Autodesk Fusion 360 part; units mm, degrees
(part 2 of 7)
sketch "Sketch40" plane through (0, 116.2145, -31.1396) normal (0, 0.965926, -0.258819) x (-1, 0, 0)
  line L0 (-109.8689, 117.075) -> (-111.5449, 117.075)
  arc A0 (-116.5449, 122.075) -> (-111.5449, 117.075) centre (-111.5449, 122.075) ccw
  line L1 (-116.5449, 122.075) -> (-116.5449, 197.0502)
  arc A1 (-111.5449, 202.0502) -> (-116.5449, 197.0502) centre (-111.5449, 197.0502) ccw
  line L2 (-111.5449, 202.0502) -> (-109.8689, 202.0502)
  arc A2 (-104.8689, 197.0502) -> (-109.8689, 202.0502) centre (-109.8689, 197.0502) ccw
  line L3 (-104.8689, 197.0502) -> (-104.8689, 122.075)
  arc A3 (-109.8689, 117.075) -> (-104.8689, 122.075) centre (-109.8689, 122.075) ccw
  line L4 (-35, 125) -> (-35, 117.5)
  arc A4 (-37.5, 115) -> (-35, 117.5) centre (-37.5, 117.5) ccw
  line L5 (-37.5, 115) -> (-65, 115)
  arc A5 (-70, 120) -> (-65, 115) centre (-65, 120) ccw
  line L6 (-70, 120) -> (-70, 125)
  arc A6 (-65, 130) -> (-70, 125) centre (-65, 125) ccw
  line L7 (-65, 130) -> (-40, 130)
  arc A7 (-35, 125) -> (-40, 130) centre (-40, 125) ccw
  line L8 (-95.5983, 117.0948) -> (-95.6526, 117.0948)
  arc A8 (-100.6526, 122.0948) -> (-95.6526, 117.0948) centre (-95.6526, 122.0948) ccw
  line L9 (-100.6526, 122.0948) -> (-100.6526, 154.3733)
  line L10 (-100.6526, 154.3733) -> (-90.5983, 154.3733)
  line L11 (-90.5983, 154.3733) -> (-90.5983, 122.0948)
  arc A9 (-95.5983, 117.0948) -> (-90.5983, 122.0948) centre (-95.5983, 122.0948) ccw
  arc A10 (-90.5983, 197.0502) -> (-95.5983, 202.0502) centre (-95.5983, 197.0502) ccw
  line L12 (-90.5983, 197.0502) -> (-90.5983, 159.5626)
  line L13 (-90.5983, 159.5626) -> (-100.6526, 159.5626)
  line L14 (-100.6526, 159.5626) -> (-100.6526, 197.0502)
  arc A11 (-95.6526, 202.0502) -> (-100.6526, 197.0502) centre (-95.6526, 197.0502) ccw
  line L15 (-95.6526, 202.0502) -> (-95.5983, 202.0502)
  line L16 (-37.5, 135) -> (-67.5, 135)
  arc A12 (-70, 137.5) -> (-67.5, 135) centre (-67.5, 137.5) ccw
  line L17 (-70, 137.5) -> (-70, 142.5)
  arc A13 (-67.5, 145) -> (-70, 142.5) centre (-67.5, 142.5) ccw
  line L18 (-67.5, 145) -> (-37.5, 145)
  arc A14 (-35, 142.5) -> (-37.5, 145) centre (-37.5, 142.5) ccw
  line L19 (-35, 142.5) -> (-35, 137.5)
  arc A15 (-37.5, 135) -> (-35, 137.5) centre (-37.5, 137.5) ccw
  arc A16 (-84.2974, 121.8844) -> (-80.3534, 116.9972) centre (-79.2974, 121.8844) ccw
  line L20 (-84.2974, 121.8844) -> (-84.2974, 171.0352)
  line L21 (-84.2974, 171.0352) -> (-76.4093, 171.0352)
  line L22 (-76.4093, 171.0352) -> (-76.4093, 121.8844)
  arc A17 (-80.3534, 116.9972) -> (-76.4093, 121.8844) centre (-81.4093, 121.8844) ccw
  arc A18 (-76.4093, 196.948) -> (-80.3534, 201.8353) centre (-81.4093, 196.948) ccw
  line L23 (-76.4093, 196.948) -> (-76.4093, 176.5782)
  line L24 (-76.4093, 176.5782) -> (-84.2974, 176.5782)
  line L25 (-84.2974, 176.5782) -> (-84.2974, 196.948)
  arc A19 (-80.3534, 201.8353) -> (-84.2974, 196.948) centre (-79.2974, 196.948) ccw
  line L26 (-120, 85) -> (-120, 100)
  arc A20 (-110, 110) -> (-120, 100) centre (-110, 100) ccw
  line L27 (-110, 110) -> (-61.6636, 110)
  arc A21 (-51.6636, 100) -> (-61.6636, 110) centre (-61.6636, 100) ccw
  line L28 (-51.6636, 100) -> (-51.6636, 85)
  arc A22 (-61.6636, 75) -> (-51.6636, 85) centre (-61.6636, 85) ccw
  line L29 (-61.6636, 75) -> (-110, 75)
  arc A23 (-120, 85) -> (-110, 75) centre (-110, 85) ccw
  line L30 (-45.44, 85) -> (-45.44, 100)
  arc A24 (-35.44, 110) -> (-45.44, 100) centre (-35.44, 100) ccw
  line L31 (-35.44, 110) -> (-20, 110)
  arc A25 (-10, 100) -> (-20, 110) centre (-20, 100) ccw
  line L32 (-10, 100) -> (-10, 85)
  arc A26 (-20, 75) -> (-10, 85) centre (-20, 85) ccw
  line L33 (-20, 75) -> (-35.44, 75)
  arc A27 (-45.44, 85) -> (-35.44, 75) centre (-35.44, 85) ccw
  line L34 (22.9316, 100) -> (22.9316, 85)
  arc A28 (12.9316, 75) -> (22.9316, 85) centre (12.9316, 85) ccw
  line L35 (12.9316, 75) -> (7.9281, 75)
  arc A29 (-2.0719, 85) -> (7.9281, 75) centre (7.9281, 85) ccw
  line L36 (-2.0719, 85) -> (-2.0719, 100)
  arc A30 (7.9281, 110) -> (-2.0719, 100) centre (7.9281, 100) ccw
  line L37 (7.9281, 110) -> (12.9316, 110)
  arc A31 (22.9316, 100) -> (12.9316, 110) centre (12.9316, 100) ccw
  line L38 (-40, 30) -> (-110, 30)
  arc A32 (-120, 40) -> (-110, 30) centre (-110, 40) ccw
  line L39 (-120, 40) -> (-120, 60)
  arc A33 (-110, 70) -> (-120, 60) centre (-110, 60) ccw
  line L40 (-110, 70) -> (-40, 70)
  arc A34 (-30, 60) -> (-40, 70) centre (-40, 60) ccw
  line L41 (-30, 60) -> (-30, 40)
  arc A35 (-40, 30) -> (-30, 40) centre (-40, 40) ccw
  line L42 (-10, 70) -> (10, 70)
  arc A36 (20, 60) -> (10, 70) centre (10, 60) ccw
  line L43 (20, 60) -> (20, 40)
  arc A37 (10, 30) -> (20, 40) centre (10, 40) ccw
  line L44 (10, 30) -> (-10, 30)
  arc A38 (-20, 40) -> (-10, 30) centre (-10, 40) ccw
  line L45 (-20, 40) -> (-20, 60)
  arc A39 (-10, 70) -> (-20, 60) centre (-10, 60) ccw
  ellipse E0 centre (22.741, -39.3535) end of major axis (22.741, -46.5838) minor radius 7 (22.741, -46.5838) -> (29.741, -39.3535) ccw
  line L46 (29.741, -39.3535) -> (29.741, 209.5755)
  ellipse E1 centre (22.741, 209.5755) end of major axis (22.741, 216.8058) minor radius 7 (29.741, 209.5755) -> (22.741, 216.8058) ccw
  line L47 (22.741, 216.8058) -> (-123.259, 216.8058)
  ellipse E2 centre (-123.259, 209.5755) end of major axis (-123.259, 216.8058) minor radius 7 (-123.259, 216.8058) -> (-130.259, 209.5755) ccw
  line L48 (-130.259, 209.5755) -> (-130.259, -39.3535)
  ellipse E3 centre (-123.259, -39.3535) end of major axis (-123.259, -46.5838) minor radius 7 (-130.259, -39.3535) -> (-123.259, -46.5838) ccw
  line L49 (-123.259, -46.5838) -> (22.741, -46.5838)
  line L50 (-35.9419, 179.9959) -> (-35.9419, 150.9959)
  line L51 (-35.9419, 150.9959) -> (-72.9419, 150.9959)
  line L52 (-72.9419, 150.9959) -> (-72.9419, 179.9959)
  line L53 (-72.9419, 179.9959) -> (-35.9419, 179.9959)
  line L54 (0, 145) -> (25, 155)
  line L55 (25, 155) -> (25, 160)
  line L56 (25, 160) -> (0, 150)
  line L57 (0, 150) -> (0, 145)
  line L58 (0, 155) -> (25, 165)
  line L59 (25, 165) -> (25, 170)
  line L60 (25, 170) -> (0, 160)
  line L61 (0, 160) -> (0, 155)
  line L62 (0, 165) -> (25, 175)
  line L63 (25, 175) -> (25, 180.1705)
  line L64 (0, 165) -> (0, 170)
  line L65 (0, 170) -> (25, 180.1705)
  line L66 (0, 175) -> (25, 185)
  line L67 (25, 185) -> (25, 190.1897)
  line L68 (25, 190.1897) -> (0, 180.1897)
  line L69 (0, 180.1897) -> (0, 175)
  line L70 (0, 185) -> (25, 195)
  line L71 (25, 195) -> (25, 200)
  line L72 (25, 200) -> (0, 190)
  line L73 (0, 190) -> (0, 185)
  line L74 (0, 195) -> (25, 205)
  line L75 (25, 205) -> (25, 210)
  line L76 (25, 210) -> (0, 200)
  line L77 (0, 200) -> (0, 195)
  line L78 (-5, 145) -> (-30, 150)
  line L79 (-30, 150) -> (-30, 155)
  line L80 (-30, 155) -> (-5, 150)
  line L81 (-5, 150) -> (-5, 145)
  line L82 (-5, 155) -> (-30, 160)
  line L83 (-30, 160) -> (-30, 165.149)
  line L84 (-30, 165.149) -> (-5, 160.149)
  line L85 (-5, 160.149) -> (-5, 155)
  line L86 (-5, 165) -> (-30, 170)
  line L87 (-30, 170) -> (-30, 175)
  line L88 (-30, 175) -> (-5, 170)
  line L89 (-5, 170) -> (-5, 165)
  line L90 (-5, 175) -> (-30, 180)
  line L91 (-30, 180) -> (-30, 184.9041)
  line L92 (-30, 184.9041) -> (-5, 180)
  line L93 (-5, 180) -> (-5, 175)
  line L94 (-5, 184.9041) -> (-30, 189.9041)
  line L95 (-30, 189.9041) -> (-30, 195)
  line L96 (-30, 195) -> (-5, 190)
  line L97 (-5, 184.9041) -> (-5, 190)
  line L98 (-5, 195) -> (-30, 200)
  line L99 (-30, 200) -> (-30, 205)
  line L100 (-30, 205) -> (-5, 200)
  line L101 (-5, 200) -> (-5, 195)
  constraint parallel L54 L56
  constraint parallel L56 L58
  constraint parallel L57 L59
  constraint parallel L56 L60
  constraint parallel L57 L61
  constraint parallel L60 L62
  constraint parallel L61 L63
  constraint vertical L64
  constraint parallel L62 L66
  constraint parallel L63 L67
  constraint parallel L62 L68
  constraint vertical L69
  constraint parallel L66 L70
  constraint parallel L69 L71
  constraint parallel L70 L72
  constraint parallel L71 L73
  constraint parallel L72 L74
  constraint parallel L73 L75
  constraint parallel L74 L76
  constraint parallel L75 L77
  constraint parallel L78 L82
  constraint parallel L81 L83
  constraint parallel L78 L84
  constraint parallel L82 L86
  constraint parallel L85 L87
  constraint parallel L82 L88
  constraint parallel L86 L90
  constraint parallel L89 L91
  constraint parallel L90 L94
  constraint parallel L93 L95
  constraint parallel L90 L96
  constraint parallel L96 L98
  constraint parallel L97 L99
  constraint parallel L96 L100
  constraint vertical L101
sketch "Sketch41" plane through (0, 116.2145, -31.1396) normal (0, 0.965926, -0.258819) x (-1, 0, 0)
  line L0 (25, 185) -> (0, 175)
  line L1 (0, 175) -> (0, 180.1897)
  line L2 (0, 180.1897) -> (25, 190.1897)
  line L3 (25, 190.1897) -> (25, 185)
  line L4 (-5, 190) -> (-5, 184.9041)
  line L5 (-5, 184.9041) -> (-30, 189.9041)
  line L6 (-30, 189.9041) -> (-30, 195)
  line L7 (-30, 195) -> (-5, 190)
  line L8 (-30, 150) -> (-30, 155)
  line L9 (-30, 155) -> (-5, 150)
  line L10 (-5, 150) -> (-5, 145)
  line L11 (-5, 145) -> (-30, 150)
  line L12 (-30, 160) -> (-30, 165.149)
  line L13 (-30, 165.149) -> (-5, 160.149)
  line L14 (-5, 160.149) -> (-5, 155)
  line L15 (-5, 155) -> (-30, 160)
  line L16 (-30, 200) -> (-30, 205)
  line L17 (-30, 205) -> (-5, 200)
  line L18 (-5, 200) -> (-5, 195)
  line L19 (-5, 195) -> (-30, 200)
  line L20 (25, 180.1705) -> (25, 175)
  line L21 (25, 175) -> (0, 165)
  line L22 (0, 165) -> (0, 170)
  line L23 (0, 170) -> (25, 180.1705)
  line L24 (25, 155) -> (0, 145)
  line L25 (0, 145) -> (0, 150)
  line L26 (0, 150) -> (25, 160)
  line L27 (25, 160) -> (25, 155)
  line L28 (25, 195) -> (0, 185)
  line L29 (0, 185) -> (0, 190)
  line L30 (0, 190) -> (25, 200)
  line L31 (25, 200) -> (25, 195)
  line L32 (-30, 180) -> (-30, 184.9041)
  line L33 (-30, 184.9041) -> (-5, 180)
  line L34 (-5, 180) -> (-5, 175)
  line L35 (-5, 175) -> (-30, 180)
  line L36 (-30, 170) -> (-30, 175)
  line L37 (-30, 175) -> (-5, 170)
  line L38 (-5, 170) -> (-5, 165)
  line L39 (-5, 165) -> (-30, 170)
  line L40 (25, 205) -> (0, 195)
  line L41 (0, 195) -> (0, 200)
  line L42 (0, 200) -> (25, 210)
  line L43 (25, 210) -> (25, 205)
  line L44 (25, 165) -> (0, 155)
  line L45 (0, 155) -> (0, 160)
  line L46 (0, 160) -> (25, 170)
  line L47 (25, 170) -> (25, 165)
  line L48 (-109.8689, 117.075) -> (-111.5449, 117.075)
  arc A0 (-116.5449, 122.075) -> (-111.5449, 117.075) centre (-111.5449, 122.075) ccw
  line L49 (-116.5449, 122.075) -> (-116.5449, 197.0502)
  arc A1 (-111.5449, 202.0502) -> (-116.5449, 197.0502) centre (-111.5449, 197.0502) ccw
  line L50 (-111.5449, 202.0502) -> (-109.8689, 202.0502)
  arc A2 (-104.8689, 197.0502) -> (-109.8689, 202.0502) centre (-109.8689, 197.0502) ccw
  line L51 (-104.8689, 197.0502) -> (-104.8689, 122.075)
  arc A3 (-109.8689, 117.075) -> (-104.8689, 122.075) centre (-109.8689, 122.075) ccw
  line L52 (-35, 125) -> (-35, 117.5)
  arc A4 (-37.5, 115) -> (-35, 117.5) centre (-37.5, 117.5) ccw
  line L53 (-37.5, 115) -> (-65, 115)
  arc A5 (-70, 120) -> (-65, 115) centre (-65, 120) ccw
  line L54 (-70, 120) -> (-70, 125)
  arc A6 (-65, 130) -> (-70, 125) centre (-65, 125) ccw
  line L55 (-65, 130) -> (-40, 130)
  arc A7 (-35, 125) -> (-40, 130) centre (-40, 125) ccw
  line L56 (-95.5983, 117.0948) -> (-95.6526, 117.0948)
  arc A8 (-100.6526, 122.0948) -> (-95.6526, 117.0948) centre (-95.6526, 122.0948) ccw
  line L57 (-100.6526, 122.0948) -> (-100.6526, 154.3733)
  line L58 (-100.6526, 154.3733) -> (-90.5983, 154.3733)
  line L59 (-90.5983, 154.3733) -> (-90.5983, 122.0948)
  arc A9 (-95.5983, 117.0948) -> (-90.5983, 122.0948) centre (-95.5983, 122.0948) ccw
  arc A10 (-90.5983, 197.0502) -> (-95.5983, 202.0502) centre (-95.5983, 197.0502) ccw
  line L60 (-90.5983, 197.0502) -> (-90.5983, 159.5626)
  line L61 (-90.5983, 159.5626) -> (-100.6526, 159.5626)
  line L62 (-100.6526, 159.5626) -> (-100.6526, 197.0502)
  arc A11 (-95.6526, 202.0502) -> (-100.6526, 197.0502) centre (-95.6526, 197.0502) ccw
  line L63 (-95.6526, 202.0502) -> (-95.5983, 202.0502)
  line L64 (-37.5, 135) -> (-67.5, 135)
  arc A12 (-70, 137.5) -> (-67.5, 135) centre (-67.5, 137.5) ccw
  line L65 (-70, 137.5) -> (-70, 142.5)
  arc A13 (-67.5, 145) -> (-70, 142.5) centre (-67.5, 142.5) ccw
  line L66 (-67.5, 145) -> (-37.5, 145)
  arc A14 (-35, 142.5) -> (-37.5, 145) centre (-37.5, 142.5) ccw
  line L67 (-35, 142.5) -> (-35, 137.5)
  arc A15 (-37.5, 135) -> (-35, 137.5) centre (-37.5, 137.5) ccw
  arc A16 (-84.2974, 121.8844) -> (-80.3534, 116.9972) centre (-79.2974, 121.8844) ccw
  line L68 (-84.2974, 121.8844) -> (-84.2974, 171.0352)
  line L69 (-84.2974, 171.0352) -> (-76.4093, 171.0352)
  line L70 (-76.4093, 171.0352) -> (-76.4093, 121.8844)
  arc A17 (-80.3534, 116.9972) -> (-76.4093, 121.8844) centre (-81.4093, 121.8844) ccw
  arc A18 (-76.4093, 196.948) -> (-80.3534, 201.8353) centre (-81.4093, 196.948) ccw
  line L71 (-76.4093, 196.948) -> (-76.4093, 176.5782)
  line L72 (-76.4093, 176.5782) -> (-84.2974, 176.5782)
  line L73 (-84.2974, 176.5782) -> (-84.2974, 196.948)
  arc A19 (-80.3534, 201.8353) -> (-84.2974, 196.948) centre (-79.2974, 196.948) ccw
  line L74 (-120, 85) -> (-120, 100)
  arc A20 (-110, 110) -> (-120, 100) centre (-110, 100) ccw
  line L75 (-110, 110) -> (-61.6636, 110)
  arc A21 (-51.6636, 100) -> (-61.6636, 110) centre (-61.6636, 100) ccw
  line L76 (-51.6636, 100) -> (-51.6636, 85)
  arc A22 (-61.6636, 75) -> (-51.6636, 85) centre (-61.6636, 85) ccw
  line L77 (-61.6636, 75) -> (-110, 75)
  arc A23 (-120, 85) -> (-110, 75) centre (-110, 85) ccw
  line L78 (-45.44, 85) -> (-45.44, 100)
  arc A24 (-35.44, 110) -> (-45.44, 100) centre (-35.44, 100) ccw
  line L79 (-35.44, 110) -> (-20, 110)
  arc A25 (-10, 100) -> (-20, 110) centre (-20, 100) ccw
  line L80 (-10, 100) -> (-10, 85)
  arc A26 (-20, 75) -> (-10, 85) centre (-20, 85) ccw
  line L81 (-20, 75) -> (-35.44, 75)
  arc A27 (-45.44, 85) -> (-35.44, 75) centre (-35.44, 85) ccw
  line L82 (22.9316, 100) -> (22.9316, 85)
  arc A28 (12.9316, 75) -> (22.9316, 85) centre (12.9316, 85) ccw
  line L83 (12.9316, 75) -> (7.9281, 75)
  arc A29 (-2.0719, 85) -> (7.9281, 75) centre (7.9281, 85) ccw
  line L84 (-2.0719, 85) -> (-2.0719, 100)
  arc A30 (7.9281, 110) -> (-2.0719, 100) centre (7.9281, 100) ccw
  line L85 (7.9281, 110) -> (12.9316, 110)
  arc A31 (22.9316, 100) -> (12.9316, 110) centre (12.9316, 100) ccw
  line L86 (-40, 30) -> (-110, 30)
  arc A32 (-120, 40) -> (-110, 30) centre (-110, 40) ccw
  line L87 (-120, 40) -> (-120, 60)
  arc A33 (-110, 70) -> (-120, 60) centre (-110, 60) ccw
  line L88 (-110, 70) -> (-40, 70)
  arc A34 (-30, 60) -> (-40, 70) centre (-40, 60) ccw
  line L89 (-30, 60) -> (-30, 40)
  arc A35 (-40, 30) -> (-30, 40) centre (-40, 40) ccw
  line L90 (-10, 70) -> (10, 70)
  arc A36 (20, 60) -> (10, 70) centre (10, 60) ccw
  line L91 (20, 60) -> (20, 40)
  arc A37 (10, 30) -> (20, 40) centre (10, 40) ccw
  line L92 (10, 30) -> (-10, 30)
  arc A38 (-20, 40) -> (-10, 30) centre (-10, 40) ccw
  line L93 (-20, 40) -> (-20, 60)
  arc A39 (-10, 70) -> (-20, 60) centre (-10, 60) ccw
  ellipse E0 centre (22.741, -39.3535) end of major axis (22.741, -46.5838) minor radius 7 (22.741, -46.5838) -> (29.741, -39.3535) ccw
  line L94 (29.741, -39.3535) -> (29.741, 209.5755)
  ellipse E1 centre (22.741, 209.5755) end of major axis (22.741, 216.8058) minor radius 7 (29.741, 209.5755) -> (22.741, 216.8058) ccw
  line L95 (22.741, 216.8058) -> (-123.259, 216.8058)
  ellipse E2 centre (-123.259, 209.5755) end of major axis (-123.259, 216.8058) minor radius 7 (-123.259, 216.8058) -> (-130.259, 209.5755) ccw
  line L96 (-130.259, 209.5755) -> (-130.259, -39.3535)
  ellipse E3 centre (-123.259, -39.3535) end of major axis (-123.259, -46.5838) minor radius 7 (-130.259, -39.3535) -> (-123.259, -46.5838) ccw
  line L97 (-123.259, -46.5838) -> (22.741, -46.5838)
  line L98 (-35.9419, 179.9959) -> (-35.9419, 150.9959)
  line L99 (-35.9419, 150.9959) -> (-72.9419, 150.9959)
  line L100 (-72.9419, 150.9959) -> (-72.9419, 179.9959)
  line L101 (-72.9419, 179.9959) -> (-35.9419, 179.9959)
  line L102 (-68.3957, 196.948) -> (-56.6, 196.948)
  line L103 (-55, 195.348) -> (-55, 186.6)
  line L104 (-56.6, 185) -> (-68.3957, 185)
  line L105 (-69.9957, 186.6) -> (-69.9957, 195.348)
  line L106 (-48.311, 196.948) -> (-36.6, 196.948)
  line L107 (-35, 195.348) -> (-35, 186.6)
  line L108 (-36.6, 185) -> (-48.311, 185)
  line L109 (-49.911, 186.6) -> (-49.911, 195.348)
  line L110 (-68.7895, 206.1671) -> (-56.6, 206.1671)
  line L111 (-55, 204.5671) -> (-55, 201.6)
  line L112 (-56.6, 200) -> (-68.7895, 200)
  line L113 (-70.3895, 201.6) -> (-70.3895, 204.5671)
  line L114 (-48.311, 206.2984) -> (-36.6, 206.2984)
  line L115 (-35, 204.6984) -> (-35, 201.6)
  line L116 (-36.6, 200) -> (-48.311, 200)
  line L117 (-49.911, 201.6) -> (-49.911, 204.6984)
  arc A40 (-68.7895, 206.1671) -> (-70.3895, 204.5671) centre (-68.7895, 204.5671) ccw
  arc A41 (-70.3895, 201.6) -> (-68.7895, 200) centre (-68.7895, 201.6) ccw
  arc A42 (-56.6, 200) -> (-55, 201.6) centre (-56.6, 201.6) ccw
  arc A43 (-55, 204.5671) -> (-56.6, 206.1671) centre (-56.6, 204.5671) ccw
  arc A44 (-48.311, 206.2984) -> (-49.911, 204.6984) centre (-48.311, 204.6984) ccw
  arc A45 (-49.911, 201.6) -> (-48.311, 200) centre (-48.311, 201.6) ccw
  arc A46 (-36.6, 200) -> (-35, 201.6) centre (-36.6, 201.6) ccw
  arc A47 (-35, 204.6984) -> (-36.6, 206.2984) centre (-36.6, 204.6984) ccw
  arc A48 (-35, 195.348) -> (-36.6, 196.948) centre (-36.6, 195.348) ccw
  arc A49 (-48.311, 196.948) -> (-49.911, 195.348) centre (-48.311, 195.348) ccw
  arc A50 (-49.911, 186.6) -> (-48.311, 185) centre (-48.311, 186.6) ccw
  arc A51 (-36.6, 185) -> (-35, 186.6) centre (-36.6, 186.6) ccw
  arc A52 (-56.6, 185) -> (-55, 186.6) centre (-56.6, 186.6) ccw
  arc A53 (-69.9957, 186.6) -> (-68.3957, 185) centre (-68.3957, 186.6) ccw
  arc A54 (-68.3957, 196.948) -> (-69.9957, 195.348) centre (-68.3957, 195.348) ccw
  arc A55 (-55, 195.348) -> (-56.6, 196.948) centre (-56.6, 195.348) ccw
  dimension "d130" = 1.6
  constraint horizontal L102
  constraint vertical L103
  constraint horizontal L104
  constraint vertical L105
  constraint horizontal L106
  constraint vertical L107
  constraint horizontal L108
  constraint vertical L109
  constraint horizontal L110
  constraint vertical L111
  constraint horizontal L112
  constraint vertical L113
  constraint horizontal L114
  constraint vertical L115
  constraint horizontal L116
  constraint vertical L117
  constraint tangent L110 A40
  constraint tangent L113 A40
  constraint tangent L112 A41
  constraint tangent L113 A41
  constraint equal A40 A41
  constraint tangent L111 A42
  constraint tangent L112 A42
  constraint equal A40 A42
  constraint tangent L110 A43
  constraint tangent L111 A43
  constraint equal A40 A43
  constraint tangent L114 A44
  constraint tangent L117 A44
  constraint equal A40 A44
  constraint tangent L116 A45
  constraint tangent L117 A45
  constraint equal A40 A45
  constraint tangent L115 A46
  constraint tangent L116 A46
  constraint equal A40 A46
  constraint tangent L114 A47
  constraint tangent L115 A47
  constraint equal A40 A47
  constraint tangent L106 A48
  constraint tangent L107 A48
  constraint equal A40 A48
  constraint tangent L106 A49
  constraint tangent L109 A49
  constraint equal A40 A49
  constraint tangent L108 A50
  constraint tangent L109 A50
  constraint equal A40 A50
  constraint tangent L107 A51
  constraint tangent L108 A51
  constraint equal A40 A51
  constraint tangent L103 A52
  constraint tangent L104 A52
  constraint equal A40 A52
  constraint tangent L104 A53
  constraint tangent L105 A53
  constraint equal A40 A53
  constraint tangent L102 A54
  constraint tangent L105 A54
  constraint equal A40 A54
  constraint tangent L102 A55
  constraint tangent L103 A55
  constraint equal A40 A55
  measures "d130" radius of A40
sketch "Sketch42" plane through (130.259, 0, 0) normal (1, 0, 0) x (0, 0, -1)
  line L0 (-45, 101.218) -> (-45, 110)
  line L1 (-45, 110) -> (-6.7003, 110)
  line L2 (-6.7003, 110) -> (-6.7003, 101.218)
  line L3 (-6.7003, 101.218) -> (-45, 101.218)
  line L4 (69.1009, 100.1665) -> (69.1521, 106.0291)
  line L5 (69.1521, 106.0291) -> (-171.2948, 170.4566)
  line L6 (-171.2948, 170.4566) -> (-171.8899, 102.2696)
  line L7 (-171.8899, 102.2696) -> (69.1009, 100.1665)
  line L8 (-161.2986, 157.4875) -> (-51.9598, 127.9462)
  line L9 (-50.7621, 125.8617) -> (-51.5882, 122.8043)
  line L10 (-53.6727, 121.6065) -> (-163.2369, 151.2087)
  line L11 (-164.3976, 153.4127) -> (-163.3462, 156.4092)
  arc A0 (-161.2986, 157.4875) -> (-163.3462, 156.4092) centre (-161.7421, 155.8464) ccw
  arc A1 (-164.3976, 153.4127) -> (-163.2369, 151.2087) centre (-162.7935, 152.8499) ccw
  arc A2 (-53.6727, 121.6065) -> (-51.5882, 122.8043) centre (-53.2293, 123.2477) ccw
  arc A3 (-50.7621, 125.8617) -> (-51.9598, 127.9462) centre (-52.4033, 126.3051) ccw
  line L12 (-161.5596, 143.8754) -> (-53.7157, 116.9071)
  line L13 (-52.6971, 115.2093) -> (-53.3374, 112.6488)
  line L14 (-55.0352, 111.6302) -> (-163.1254, 138.6601)
  line L15 (-164.1052, 140.4863) -> (-163.2187, 142.9853)
  arc A4 (-161.5596, 143.8754) -> (-163.2187, 142.9853) centre (-161.8993, 142.5172) ccw
  arc A5 (-164.1052, 140.4863) -> (-163.1254, 138.6601) centre (-162.7858, 140.0182) ccw
  arc A6 (-55.0352, 111.6302) -> (-53.3374, 112.6488) centre (-54.6956, 112.9884) ccw
  arc A7 (-52.6971, 115.2093) -> (-53.7157, 116.9071) centre (-54.0553, 115.5489) ccw
  line L16 (-161.9239, 132.0685) -> (-54.4887, 107.4182)
  line L17 (-53.7377, 106.2199) -> (-54.0929, 104.6716)
  line L18 (-55.2912, 103.9206) -> (-162.9172, 128.6146)
  line L19 (-163.6336, 129.9305) -> (-163.0875, 131.435)
  arc A8 (-161.9239, 132.0685) -> (-163.0875, 131.435) centre (-162.1475, 131.0938) ccw
  arc A9 (-163.6336, 129.9305) -> (-162.9172, 128.6146) centre (-162.6936, 129.5893) ccw
  arc A10 (-55.2912, 103.9206) -> (-54.0929, 104.6716) centre (-55.0676, 104.8952) ccw
  arc A11 (-53.7377, 106.2199) -> (-54.4887, 107.4182) centre (-54.7123, 106.4435) ccw
  line L20 (-85.206, 106.0215) -> (-85.5559, 104.3593)
  line L21 (-161.6739, 120.4346) -> (-161.2418, 122.0794)
  arc A12 (-160.0686, 122.8039) -> (-161.2418, 122.0794) centre (-160.2746, 121.8254) ccw
  arc A13 (-161.6739, 120.4346) -> (-160.9127, 119.202) centre (-160.7067, 120.1805) ccw
  arc A14 (-86.7405, 103.5868) -> (-85.5559, 104.3593) centre (-86.5345, 104.5653) ccw
  arc A15 (-85.206, 106.0215) -> (-85.9786, 107.206) centre (-86.1846, 106.2275) ccw
  dimension "d133" = 1.7
  dimension "d134" = 1.4
  dimension "d135" = 1
  dimension "d136" = 1
  constraint perpendicular L8 L9
  constraint perpendicular L9 L10
  constraint tangent L11 A0
  constraint tangent L8 A0
  constraint tangent L10 A1
  constraint tangent L11 A1
  constraint equal A0 A1
  constraint tangent L10 A2
  constraint tangent L9 A2
  constraint equal A0 A2
  constraint tangent L8 A3
  constraint tangent L9 A3
  constraint equal A0 A3
  constraint perpendicular L12 L13
  constraint perpendicular L13 L14
  constraint tangent L12 A4
  constraint tangent L15 A4
  constraint tangent L14 A5
  constraint tangent L15 A5
  constraint equal A4 A5
  constraint tangent L14 A6
  constraint tangent L13 A6
  constraint equal A4 A6
  constraint tangent L12 A7
  constraint tangent L13 A7
  constraint equal A4 A7
  constraint perpendicular L16 L17
  constraint perpendicular L17 L18
  constraint tangent L16 A8
  constraint tangent L19 A8
  constraint tangent L18 A9
  constraint tangent L19 A9
  constraint equal A8 A9
  constraint tangent L18 A10
  constraint tangent L17 A10
  constraint equal A8 A10
  constraint tangent L16 A11
  constraint tangent L17 A11
  constraint equal A8 A11
  constraint tangent L21 A12
  constraint tangent L21 A13
  constraint equal A12 A13
  constraint tangent L20 A14
  constraint equal A12 A14
  constraint tangent L20 A15
  constraint equal A12 A15
  measures "d133" radius of A0
  measures "d134" radius of A4
  measures "d135" radius of A8
  measures "d136" radius of A12
sketch "Sketch43" plane through (0, 113.3167, -30.3631) normal (0, -0.965926, 0.258819) x (1, 0, 0)
  line L0 (35.9419, 150.9959) -> (35.9419, 179.9959)
  line L1 (35.9419, 179.9959) -> (72.9419, 179.9959)
  line L2 (72.9419, 179.9959) -> (72.9419, 150.9959)
  line L3 (72.9419, 150.9959) -> (35.9419, 150.9959)
  line L4 (-26.741, -44.2609) -> (127.259, -44.2609)
  line L5 (127.259, -44.2609) -> (127.259, 212.9313)
  line L6 (127.259, 212.9313) -> (-26.741, 212.9313)
  line L7 (-26.741, 212.9313) -> (-26.741, -44.2609)
  line L8 (29.2674, 103.4985) -> (48.7311, 103.4985)
  line L9 (48.7311, 103.4985) -> (48.7311, 74.7843)
  line L10 (48.7311, 74.7843) -> (29.2674, 74.7843)
  line L11 (29.2674, 74.7843) -> (29.2674, 103.4985)
  constraint horizontal L8
  constraint vertical L9
  constraint horizontal L10
  constraint vertical L11
sketch "Sketch44" plane through (0, 60, 0) normal (0, -1, 0) x (1, 0, 0)
  line L0 (-24.7646, 93.5608) -> (-24.7646, 143.5608)
  line L1 (-24.7646, 143.5608) -> (-4.7646, 143.5608)
  line L2 (-4.7646, 143.5608) -> (-4.7646, 93.5608)
  line L3 (-4.7646, 93.5608) -> (-24.7646, 93.5608)
  line L4 (104.6989, 93.7931) -> (104.6989, 143.7931)
  line L5 (104.6989, 143.7931) -> (124.6989, 143.7931)
  line L6 (124.6989, 143.7931) -> (124.6989, 93.7931)
  line L7 (124.6989, 93.7931) -> (104.6989, 93.7931)
  line L8 (-24.5171, -45.8743) -> (-24.5171, 4.1257)
  line L9 (-24.5171, 4.1257) -> (-4.5171, 4.1257)
  line L10 (-4.5171, 4.1257) -> (-4.5171, -45.8743)
  line L11 (-4.5171, -45.8743) -> (-24.5171, -45.8743)
  line L12 (123.4565, 4.1404) -> (123.4565, -45.8596)
  line L13 (123.4565, -45.8596) -> (103.4565, -45.8596)
  line L14 (103.4565, -45.8596) -> (103.4565, 4.1404)
  line L15 (103.4565, 4.1404) -> (123.4565, 4.1404)
  line L16 (110.5201, 150.9612) -> (110.5201, 145.9612)
  line L17 (110.5201, 145.9612) -> (105.5201, 145.9612)
  line L18 (105.5201, 145.9612) -> (105.5201, 150.9612)
  line L19 (105.5201, 150.9612) -> (110.5201, 150.9612)
  line L20 (-12.4226, 146.4275) -> (-17.4226, 146.4275)
  line L21 (-17.4226, 146.4275) -> (-17.4226, 151.4275)
  line L22 (-17.4226, 151.4275) -> (-12.4226, 151.4275)
  line L23 (-12.4226, 151.4275) -> (-12.4226, 146.4275)
  arc A0 (-30, -73) -> (-23, -80) centre (-23, -73) ccw
  line L24 (-23, -80) -> (123, -80)
  arc A1 (123, -80) -> (130, -73) centre (123, -73) ccw
  line L25 (130, -73) -> (130, 173)
  arc A2 (130, 173) -> (123, 180) centre (123, 173) ccw
  line L26 (123, 180) -> (-23, 180)
  arc A3 (-23, 180) -> (-30, 173) centre (-23, 173) ccw
  line L27 (-30, 173) -> (-30, -73)
  circle A4 centre (-7.4651, 81.8749) radius 2.5
  circle A5 centre (17.1849, 83.771) radius 2.5
  circle A6 centre (-6.28, 71.446) radius 2.5
  circle A7 centre (6.519, 71.9201) radius 2.5
  circle A8 centre (18.844, 72.3941) radius 2.5
  circle A9 centre (4.6229, 82.3489) radius 2.5
  circle A10 centre (-5.0949, 59.5951) radius 2.5
  circle A11 centre (20, 60) radius 2.5
  circle A12 centre (7.2301, 59.8321) radius 2.5
  circle A13 centre (111.307, 87.4438) radius 2.5
  circle A14 centre (97.1273, 86.7053) radius 2.5
  circle A15 centre (84.1293, 86.4099) radius 2.5
  circle A16 centre (112, 76) radius 2.5
  circle A17 centre (97.8486, 75.6535) radius 2.5
  circle A18 centre (85, 75) radius 2.5
  circle A19 centre (98.0745, 63.6809) radius 2.5
  circle A20 centre (112.5319, 63.9068) radius 2.5
  circle A21 centre (85.1983, 62.7773) radius 2.5
  point P0 (110.9162, 104.3617)
  point P1 (97.8486, 75.6535)
  dimension "d139" = 5
  dimension "d141" = 5
  dimension "d142" = 5
  dimension "d143" = 5
  dimension "d144" = 5
  dimension "d145" = 5
  dimension "d146" = 5
  dimension "d147" = 5
  dimension "d148" = 5
  dimension "d149" = 5
  dimension "d150" = 5
  dimension "d151" = 5
  dimension "d152" = 5
  dimension "d153" = 5
  dimension "d154" = 5
  dimension "d155" = 5
  dimension "d156" = 5
  dimension "d157" = 5
  constraint coincident P1 A17.centre
  measures "d139" diameter of A4
  measures "d141" diameter of A5
  measures "d142" diameter of A6
  measures "d143" diameter of A7
  measures "d144" diameter of A8
  measures "d145" diameter of A9
  measures "d146" diameter of A10
  measures "d147" diameter of A11
  measures "d148" diameter of A12
  measures "d149" diameter of A13
  measures "d150" diameter of A14
  measures "d151" diameter of A15
  measures "d152" diameter of A16
  measures "d153" diameter of A17
  measures "d154" diameter of A18
  measures "d155" diameter of A19
  measures "d156" diameter of A20
  measures "d157" diameter of A21
extrude "Extrude10" cut sketch "Sketch44" against normal blind 4 contours A4 | A5 | A6 | A7 | A8 | A9 | A10 | A11 | A12 | A13 | A14 | A15 | A16 | A17 | A18 | A19 | A20 | A21 bodies 2 in component "base"
sketch "Sketch45" plane through (0, 115.7315, -31.0102) normal (0, 0.965926, -0.258819) x (-1, 0, 0)
  arc A0 (20, 60) -> (10, 70) centre (10, 60) ccw
  line L0 (10, 70) -> (-10, 70)
  arc A1 (-10, 70) -> (-20, 60) centre (-10, 60) ccw
  line L1 (-20, 60) -> (-20, 40)
  arc A2 (-20, 40) -> (-10, 30) centre (-10, 40) ccw
  line L2 (-10, 30) -> (10, 30)
  arc A3 (10, 30) -> (20, 40) centre (10, 40) ccw
  line L3 (20, 40) -> (20, 60)
  line L4 (-15.3325, 68.4596) -> (-2, 54)
  line L5 (-2, 54) -> (-2, 70)
  line L6 (1, 70) -> (1, 56)
  line L7 (1, 56) -> (10.6758, 69.9771)
  line L8 (13.7877, 69.2549) -> (2, 54)
  line L9 (2, 54) -> (20, 58)
  line L10 (20, 54.6117) -> (2, 52)
  line L11 (2, 52) -> (20, 42)
  line L12 (19.651, 37.3811) -> (1, 49)
  line L13 (1, 49) -> (8, 30)
  line L14 (-18, 66) -> (-2, 52)
  line L15 (-2, 52) -> (-20, 50)
  line L16 (-20, 47) -> (-2, 49)
  line L17 (-2, 49) -> (-18.606, 34.9072)
  line L18 (-16.5714, 32.4623) -> (-1.1201, 45.5753)
  line L19 (-1.1201, 45.5753) -> (-2, 30)
  line L20 (5, 30) -> (1, 44)
  line L21 (1, 44) -> (1, 30)
  constraint coincident A1 L4.start
  constraint coincident L0 L5.end
  constraint perpendicular L0 L5
  constraint coincident L0 L6.start
  constraint perpendicular L0 L6
  constraint coincident A0 L7.end
  constraint coincident A0 L8.start
  constraint coincident L3 L9.end
  constraint coincident L3 L10.start
  constraint coincident L3 L11.end
  constraint coincident A3 L12.start
  constraint coincident L2 L13.end
  constraint coincident A1 L14.start
  constraint midpoint L1 L15.end
  constraint coincident L1 L16.start
  constraint parallel L15 L16
  constraint coincident A2 L17.end
  constraint coincident A2 L18.start
  constraint parallel L17 L18
  constraint coincident L2 L19.end
  constraint coincident L2 L20.start
  constraint coincident L2 L21.end
  constraint perpendicular L2 L21
sketch "Sketch46" plane through (0, 115.0071, -30.8161) normal (0, 0.965926, -0.258819) x (-1, 0, 0)
  arc A0 (-35.44, 110) -> (-45.44, 100) centre (-35.44, 100) ccw
  line L0 (-45.44, 100) -> (-45.44, 85)
  arc A1 (-45.44, 85) -> (-35.44, 75) centre (-35.44, 85) ccw
  line L1 (-35.44, 75) -> (-20, 75)
  arc A2 (-20, 75) -> (-10, 85) centre (-20, 85) ccw
  line L2 (-10, 85) -> (-10, 100)
  arc A3 (-10, 100) -> (-20, 110) centre (-20, 100) ccw
  line L3 (-20, 110) -> (-35.44, 110)
  circle A4 centre (-25, 90) radius 1.9713
  circle A5 centre (-30, 106) radius 1.9713
  circle A6 centre (-24, 106) radius 1.9713
  circle A7 centre (-19, 106) radius 1.9713
  circle A8 centre (-42, 101) radius 1.9713
  circle A9 centre (-36.1793, 100.5172) radius 1.9713
  circle A10 centre (-30.4049, 100.2983) radius 1.9713
  circle A11 centre (-24.3835, 100.0852) radius 1.9713
  circle A12 centre (-19, 100) radius 1.9713
  circle A13 centre (-42.5204, 95.2418) radius 1.9713
  circle A14 centre (-37, 95) radius 1.9713
  circle A15 centre (-31, 95) radius 1.9713
  circle A16 centre (-25, 95) radius 1.9713
  circle A17 centre (-19, 95) radius 1.9713
  circle A18 centre (-13.3531, 100.0319) radius 1.9713
  circle A19 centre (-13.5857, 94.6556) radius 1.9713
  circle A20 centre (-42, 90) radius 1.9713
  circle A21 centre (-37, 90) radius 1.9713
  circle A22 centre (-31, 90) radius 1.9713
  circle A23 centre (-19, 90) radius 1.9713
  circle A24 centre (-13.4258, 89.6999) radius 1.9713
  circle A25 centre (-36.1066, 106) radius 1.9713
  circle A26 centre (-42.254, 84.5844) radius 1.9713
  circle A27 centre (-36.3925, 84.4245) radius 1.9713
  circle A28 centre (-30.6908, 84.4778) radius 1.9713
  circle A29 centre (-25.2555, 84.4245) radius 1.9713
  circle A30 centre (-19.2874, 84.5311) radius 1.9713
  circle A31 centre (-14, 85) radius 1.9713
  circle A32 centre (-36.6394, 78.7704) radius 1.9713
  circle A33 centre (-31.3108, 78.504) radius 1.9713
  circle A34 centre (-25.9288, 78.504) radius 1.9713
  circle A35 centre (-20.0672, 78.504) radius 1.9713
sketch "Sketch47" plane through (0, 115.0071, -30.8161) normal (0, 0.965926, -0.258819) x (-1, 0, 0)
  arc A0 (12.9316, 75) -> (22.9316, 85) centre (12.9316, 85) ccw
  line L0 (22.9316, 85) -> (22.9316, 100)
  arc A1 (22.9316, 100) -> (12.9316, 110) centre (12.9316, 100) ccw
  line L1 (12.9316, 110) -> (7.9281, 110)
  arc A2 (7.9281, 110) -> (-2.0719, 100) centre (7.9281, 100) ccw
  line L2 (-2.0719, 100) -> (-2.0719, 85)
  arc A3 (-2.0719, 85) -> (7.9281, 75) centre (7.9281, 85) ccw
  line L3 (7.9281, 75) -> (12.9316, 75)
  line L4 (12, 108) -> (20.6022, 103.8891)
  line L5 (20.6022, 103.8891) -> (20.1096, 102.8584)
  line L6 (20.1096, 102.8584) -> (9.8809, 107.7465)
  line L7 (9.8809, 107.7465) -> (10.3372, 108.7014)
  line L8 (10.3372, 108.7014) -> (12, 108)
  line L9 (21, 101) -> (11.1686, 105.6983)
  line L10 (11.1686, 105.6983) -> (10.5788, 104.464)
  line L11 (10.5788, 104.464) -> (20.5406, 99.7034)
  line L12 (20.5406, 99.7034) -> (21, 101)
  line L13 (11.4135, 102.5204) -> (20.7703, 98.049)
  line L14 (20.7703, 98.049) -> (20.2687, 96.9993)
  line L15 (20.2687, 96.9993) -> (10.9117, 101.4709)
  line L16 (10.9117, 101.4709) -> (11.4135, 102.5204)
  line L17 (11.4135, 99.6967) -> (20.5195, 95.3424)
  line L18 (20.5195, 95.3424) -> (20.0533, 94.3675)
  line L19 (20.0533, 94.3675) -> (10.9611, 98.7152)
  line L20 (10.9611, 98.7152) -> (11.4135, 99.6967)
  line L21 (12, 97) -> (20.7749, 92.8041)
  line L22 (20.7749, 92.8041) -> (20.2469, 91.6998)
  line L23 (20.2469, 91.6998) -> (11.4135, 95.9237)
  line L24 (11.4135, 95.9237) -> (12, 97)
  line L25 (12, 94) -> (20.5109, 89.9303)
  line L26 (20.5109, 89.9303) -> (20.09, 89.05)
  line L27 (20.09, 89.05) -> (11.5547, 93.1314)
  line L28 (11.5547, 93.1314) -> (12, 94)
  line L29 (12.5784, 91.1901) -> (21, 87)
  line L30 (21, 87) -> (20.4293, 85.8529)
  line L31 (20.4293, 85.8529) -> (11.9774, 90.058)
  line L32 (11.9774, 90.058) -> (12.5784, 91.1901)
  line L33 (12.5784, 87.9555) -> (20.7146, 83.9074)
  line L34 (20.7146, 83.9074) -> (20.132, 82.7363)
  line L35 (20.132, 82.7363) -> (12, 87)
  line L36 (12, 87) -> (12.5784, 87.9555)
  line L37 (10.2226, 106.0843) -> (9.6237, 104.8556)
  line L38 (9.6237, 104.8556) -> (4.1192, 107.5391)
  line L39 (4.1192, 107.5391) -> (4.7076, 108.7462)
  line L40 (4.7076, 108.7462) -> (10.2226, 106.0843)
  line L41 (10.6223, 102.9389) -> (10.1031, 101.8524)
  line L42 (10.1031, 101.8524) -> (2.0211, 106.0857)
  line L43 (2.0211, 106.0857) -> (2.5, 107)
  line L44 (2.5, 107) -> (10.6223, 102.9389)
  line L45 (10.1903, 100.2152) -> (9.6698, 99.1742)
  line L46 (9.6698, 99.1742) -> (0.2801, 104.1918)
  line L47 (0.8839, 105.1912) -> (0.2801, 104.1918)
  line L48 (0.8839, 105.1912) -> (10.1903, 100.2152)
  line L49 (10.7329, 97.6028) -> (10.1903, 96.5875)
  line L50 (10.1903, 96.5875) -> (-0.4134, 102.2538)
  line L51 (-0.4134, 102.2538) -> (0.0768, 103.1712)
  line L52 (0.0768, 103.1712) -> (10.7329, 97.6028)
  line L53 (11, 94.5) -> (10.4828, 93.4183)
  line L54 (10.4828, 93.4183) -> (-0.9775, 99.4069)
  line L55 (-0.9775, 99.4069) -> (-0.2802, 100.387)
  line L56 (-0.2802, 100.387) -> (11, 94.5)
  line L57 (11.2488, 91.685) -> (10.6398, 90.4113)
  line L58 (10.6398, 90.4113) -> (-0.9465, 96.7133)
  line L59 (-0.9465, 96.7133) -> (-0.0819, 97.8054)
  line L60 (-0.0819, 97.8054) -> (11.2488, 91.685)
  line L61 (11.2488, 88.6134) -> (10.6408, 87.4498)
  line L62 (10.6408, 87.4498) -> (-0.781, 93.4183)
  line L63 (-0.781, 93.4183) -> (0, 94.5)
  line L64 (0, 94.5) -> (11.2488, 88.6134)
  line L65 (20, 81) -> (12.3888, 85.1113)
  line L66 (12.3888, 85.1113) -> (11.7297, 83.891)
  line L67 (11.7297, 83.891) -> (19.4412, 79.7255)
  line L68 (19.4412, 79.7255) -> (20, 81)
  line L69 (18.5, 79) -> (17.7795, 77.6662)
  line L70 (17.7795, 77.6662) -> (11.6076, 81)
  line L71 (11.6076, 81) -> (12.2776, 82.2404)
  line L72 (12.2776, 82.2404) -> (18.5, 79)
  line L73 (11, 86) -> (10.195, 84.4617)
  line L74 (10.195, 84.4617) -> (-0.5965, 90.4341)
  line L75 (-0.5965, 90.4341) -> (0.0248, 91.5567)
  line L76 (0.0248, 91.5567) -> (11, 86)
  line L77 (10.9448, 82.73) -> (10.3359, 81.6299)
  line L78 (10.3359, 81.6299) -> (-0.2858, 87.5083)
  line L79 (-0.2858, 87.5083) -> (0.2276, 88.436)
  line L80 (0.2276, 88.436) -> (10.9448, 82.73)
  line L81 (12, 79) -> (15.7775, 76.9094)
  line L82 (15.284, 75.8017) -> (15.7775, 76.9094)
  line L83 (15.284, 75.8017) -> (11.3938, 77.9547)
  line L84 (11.3938, 77.9547) -> (12, 79)
  line L85 (10.3459, 78.4774) -> (10.9552, 79.5783)
  line L86 (10.9552, 79.5783) -> (0.9602, 85.1098)
  line L87 (0.9602, 85.1098) -> (0.3657, 84.0356)
  line L88 (0.3657, 84.0356) -> (10.3459, 78.4774)
  line L89 (1.3959, 81.7618) -> (10, 77)
  line L90 (9.5, 76) -> (10, 77)
  line L91 (9.5, 76) -> (0.9468, 80.7336)
  line L92 (1.3959, 81.7618) -> (0.9468, 80.7336)
  constraint perpendicular L4 L5
  constraint perpendicular L5 L6
  constraint perpendicular L6 L7
  constraint perpendicular L7 L9
  constraint perpendicular L4 L10
  constraint perpendicular L7 L11
  constraint parallel L9 L13
  constraint perpendicular L13 L14
  constraint perpendicular L14 L15
  constraint perpendicular L16 L17
  constraint perpendicular L17 L18
  constraint perpendicular L18 L19
  constraint perpendicular L18 L21
  constraint perpendicular L21 L22
  constraint perpendicular L22 L23
  constraint parallel L21 L25
  constraint perpendicular L21 L26
  constraint perpendicular L26 L27
  constraint perpendicular L29 L30
  constraint perpendicular L30 L31
  constraint perpendicular L30 L33
  constraint perpendicular L31 L34
  constraint perpendicular L37 L38
  constraint perpendicular L38 L39
  constraint perpendicular L11 L41
  constraint perpendicular L42 L43
  constraint perpendicular L46 L49
  constraint perpendicular L49 L50
  constraint perpendicular L50 L51
  constraint perpendicular L27 L53
  constraint parallel L52 L54
  constraint perpendicular L25 L57
  constraint perpendicular L54 L61
  constraint perpendicular L61 L62
  constraint parallel L60 L65
  constraint perpendicular L65 L66
  constraint perpendicular L66 L67
  constraint perpendicular L65 L69
  constraint perpendicular L69 L70
  constraint perpendicular L70 L71
  constraint perpendicular L64 L73
  constraint perpendicular L74 L75
  constraint perpendicular L74 L77
  constraint perpendicular L77 L78
  constraint perpendicular L78 L79
  constraint perpendicular L77 L81
  constraint parallel L81 L83
  constraint perpendicular L81 L85
  constraint perpendicular L86 L87
  constraint perpendicular L87 L89
  constraint perpendicular L87 L91
sketch "Sketch48" plane through (0, 115.7315, -31.0102) normal (0, 0.965926, -0.258819) x (-1, 0, 0)
  arc A0 (-120, 40) -> (-110, 30) centre (-110, 40) ccw
  line L0 (-110, 30) -> (-40, 30)
  arc A1 (-40, 30) -> (-30, 40) centre (-40, 40) ccw
  line L1 (-30, 40) -> (-30, 60)
  arc A2 (-30, 60) -> (-40, 70) centre (-40, 60) ccw
  line L2 (-40, 70) -> (-110, 70)
  arc A3 (-110, 70) -> (-120, 60) centre (-110, 60) ccw
  line L3 (-120, 60) -> (-120, 40)
  line L4 (-97.4318, 70) -> (-120, 50)
  line L5 (-120, 42) -> (-87, 70)
  line L6 (-87, 70) -> (-97.4318, 70)
  line L7 (-120, 42) -> (-120, 50)
  line L8 (-87, 70) -> (-97.4318, 70)
  line L9 (-118, 34) -> (-75.5714, 70)
  line L10 (-65, 70) -> (-111.9229, 30.1866)
  line L11 (-55, 70) -> (-98, 30)
  line L12 (-86, 30) -> (-43, 70)
  line L13 (-32.9289, 67.0711) -> (-72.7803, 30)
  line L14 (-61, 30) -> (-30, 58.8372)
  line L15 (-30, 50) -> (-52, 30)
  line L16 (-40, 30) -> (-30.0261, 39.2781)
  line L17 (-120, 57) -> (-104, 70)
  constraint coincident L2 L4.start
  constraint midpoint L3 L4.end
  constraint coincident L3 L5.start
  constraint coincident L2 L5.end
  constraint coincident A0 L9.start
  constraint coincident L2 L9.end
  constraint parallel L5 L9
  constraint coincident L2 L10.start
  constraint coincident A0 L10.end
  constraint parallel L9 L10
  constraint coincident L2 L11.start
  constraint coincident L0 L11.end
  constraint coincident L0 L12.start
  constraint coincident L2 L12.end
  constraint parallel L11 L12
  constraint midpoint A2 L13.start
  constraint coincident L0 L13.end
  constraint parallel L12 L13
  constraint coincident L0 L14.start
  constraint coincident L1 L14.end
  constraint parallel L13 L14
  constraint coincident L1 L15.start
  constraint coincident L0 L15.end
  constraint midpoint L1 L15.start
  constraint coincident L0.end A1.start
  constraint coincident A1 L16.end
  constraint parallel L13 L16
  constraint coincident L3 L17.start
  constraint coincident L2 L17.end